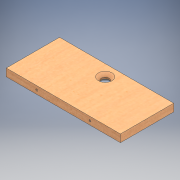
# Autodesk Inventor part: cathetherEntry
Saved by Autodesk Inventor 2018 (Build 220112000, 112)
## iProperties
Created: 2019-05-10
Part Number: cathetherEntry
Material: Generic
Document SubType Name: Modeling
Designer: aal_9
Density: 1 g/cm^3
Appearance: Default
Author: aal_9
Autodesk Inventor part; units mm, degrees
ref_plane "YZ Plane" through (0, 0, 0) normal (1, 0, 0) x (0, 1, 0)
ref_plane "XZ Plane" through (0, 0, 0) normal (0, 1, 0) x (-1, 0, 0)
ref_plane "XY Plane" through (0, 0, 0) normal (0, 0, 1) x (1, 0, 0)
sketch "Sketch1" plane through (0, 0, 0) normal (0, 1, 0) x (-1, 0, 0)
  line L0 (0, 0) -> (150, 0)
  line L1 (150, 0) -> (150, -10)
  line L2 (150, -10) -> (0, -10)
  line L3 (0, -10) -> (0, 0)
  dimension "d0" = 150
  dimension "d1" = 10
  constraints: 8 end point, 2 parallel, 1 horizontal, 1 perpendicular
  measures "d0" distance of L1.end L2.end
  measures "d1" distance of L0.end L1.end
extrude "Extrusion1" add sketch "Sketch1" along normal blind 70
sketch "Sketch2" plane through (-150, 0, 0) normal (0, 0, 1) x (1, 0, 0)
  line L0 (0, 70) -> (150, 70) projected
  line L1 (150, 0) -> (0, 0) projected
  line L2 (0, 0) -> (0, 70) projected
  point P0 (75, 55)
  dimension "d5" = 55
  dimension "d6" = 75
  measures "d5" distance from line of L1 point (75, 55)
  measures "d6" distance from line of L2 point (75, 55)
hole "Hole1" at (-75, 55, 0) direction (0, 0, -1) diameter 10 depth 10 tip angle 118
chamfer "Chamfer1" distance 4 angle 45 1 edges at (-75, 60, 0)
sketch "Sketch3" plane through (0, 0, 0) normal (0, -1, 0) x (1, 0, 0)
  line L0 (0, 0) -> (-150, 0) projected
  line L1 (-150, 0) -> (-150, -10) projected
  line L2 (0, -10) -> (0, 0) projected
  point P0 (-40, -5)
  point P1 (-110, -5)
  dimension "d18" = 5
  dimension "d19" = 5
  dimension "d20" = 40
  dimension "d21" = 40
  measures "d18" distance from line of L0 point (-40, -5)
  measures "d19" distance from line of L0 point (-110, -5)
  measures "d20" distance from line of L1 point (-110, -5)
  measures "d21" distance from line of L2 point (-40, -5)
hole "Hole2" at (-40, 0, -5) at (-110, 0, -5) direction (0, 1, 0) diameter 2.459 depth 10 tip angle 118 thread size "M3x0.5" class "6H" standard "ANSI Metric M Profile"
chamfer "Chamfer2" distance 4 angle 45 1 edges at (-75, 60, -10)
body "Solid1"
